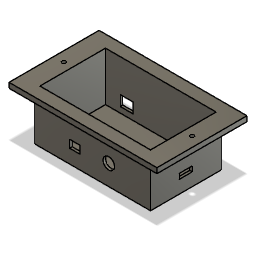
Casing light game v8 (Autodesk Fusion 360 design; units mm, degrees)
Autodesk Fusion 360 part; units mm, degrees
sketch "Sketch1" plane through (0, 0, 0) normal (0, 1, 0) x (1, 0, 0)
  line L0 (57.15, -34.925) -> (-57.15, -34.925)
  line L1 (-57.15, -34.925) -> (-57.15, 34.925)
  line L2 (-57.15, 34.925) -> (57.15, 34.925)
  line L3 (57.15, 34.925) -> (57.15, -34.925)
  line L4 (57.15, -34.925) -> (-57.15, 34.925) construction
  line L5 (-57.15, -34.925) -> (57.15, 34.925) construction
  dimension "d1" = 114.3
  dimension "d2" = 69.85
  constraint horizontal L0
  constraint perpendicular L0 L1
  constraint parallel L0 L2
  constraint parallel L1 L3
  constraint coincident L4 origin
  constraint coincident L5 origin
  measures "d1" distance of L1.end L2.end
  measures "d2" distance of L0.end L1.end
extrude "Extrude1" add sketch "Sketch1" along normal blind 44.45
sketch "Sketch10" plane through (0, 44.45, 0) normal (0, 1, 0) x (-1, 0, 0)
  line L0 (-57.15, -34.925) -> (57.15, -34.925)
  line L1 (57.15, -34.925) -> (57.15, 34.925)
  line L2 (57.15, 34.925) -> (-57.15, 34.925)
  line L3 (-57.15, 34.925) -> (-57.15, -34.925)
  line L4 (-73.025, 44.45) -> (73.025, 44.45)
  line L5 (73.025, 44.45) -> (73.025, -44.45)
  line L6 (73.025, -44.45) -> (-73.025, -44.45)
  line L7 (-73.025, -44.45) -> (-73.025, 44.45)
  line L8 (-73.025, 44.45) -> (73.025, -44.45) construction
  line L9 (73.025, 44.45) -> (-73.025, -44.45) construction
  dimension "d55" = 146.05
  dimension "d56" = 88.9
  constraint horizontal L4
  constraint perpendicular L4 L5
  constraint parallel L4 L6
  constraint parallel L5 L7
  constraint coincident L8 origin
  constraint coincident L9 origin
  measures "d55" distance of L5.end L6.end
  measures "d56" distance of L4.end L5.end
extrude "Extrude14" add sketch "Sketch10" along normal blind 5.08 contours L0 L1 L2 L3 | L4 L5 L6 L7
sketch "Sketch11" plane through (0, 49.53, 0) normal (0, 1, 0) x (-1, 0, 0)
  line L0 (-73.025, -44.45) -> (73.025, -44.45)
  line L1 (73.025, -44.45) -> (73.025, 44.45)
  line L2 (73.025, 44.45) -> (-73.025, 44.45)
  line L3 (-73.025, 44.45) -> (-73.025, -44.45)
  line L4 (57.15, -34.925) -> (-57.15, -34.925)
  line L5 (-57.15, -34.925) -> (-57.15, 34.925)
  line L6 (-57.15, 34.925) -> (57.15, 34.925)
  line L7 (57.15, 34.925) -> (57.15, -34.925)
  line L8 (63.5, -38.1) -> (-63.5, -38.1)
  line L9 (-63.5, -38.1) -> (-63.5, 38.1)
  line L10 (-63.5, 38.1) -> (63.5, 38.1)
  line L11 (63.5, 38.1) -> (63.5, -38.1)
  line L12 (63.5, -38.1) -> (-63.5, 38.1) construction
  line L13 (-63.5, -38.1) -> (63.5, 38.1) construction
  dimension "d61" = 127
  dimension "d62" = 76.2
  constraint horizontal L8
  constraint perpendicular L8 L9
  constraint parallel L8 L10
  constraint parallel L9 L11
  constraint coincident L12 origin
  constraint coincident L13 origin
  measures "d61" distance of L8.start L8.end
  measures "d62" distance of L8.start L10.end
sketch "Sketch27" plane through (0, 49.53, 0) normal (0, 1, 0) x (-1, 0, 0)
  line L0 (-73.025, -44.45) -> (73.025, -44.45)
  line L1 (73.025, -44.45) -> (73.025, 44.45)
  line L2 (73.025, 44.45) -> (-73.025, 44.45)
  line L3 (-73.025, 44.45) -> (-73.025, -44.45)
  line L4 (57.15, -34.925) -> (-57.15, -34.925)
  line L5 (-57.15, -34.925) -> (-57.15, 34.925)
  line L6 (-57.15, 34.925) -> (57.15, 34.925)
  line L7 (57.15, 34.925) -> (57.15, -34.925)
  line L8 (-54.61, 32.385) -> (54.61, 32.385)
  line L9 (54.61, 32.385) -> (54.61, -32.385)
  line L10 (54.61, -32.385) -> (-54.61, -32.385)
  line L11 (-54.61, -32.385) -> (-54.61, 32.385)
  dimension "d89" = 2.54
extrude "Extrude22" cut sketch "Sketch27" against normal blind 48.26 contours L8 L9 L10 L11
sketch "Sketch28" plane through (0, 49.53, 0) normal (0, 1, 0) x (-1, 0, 0)
  line L0 (54.61, 32.385) -> (54.61, -32.385)
  line L1 (54.61, -32.385) -> (-54.61, -32.385)
  line L2 (-54.61, -32.385) -> (-54.61, 32.385)
  line L3 (-54.61, 32.385) -> (54.61, 32.385)
  line L4 (-73.025, -44.45) -> (73.025, -44.45)
  line L5 (73.025, -44.45) -> (73.025, 44.45)
  line L6 (73.025, 44.45) -> (-73.025, 44.45)
  line L7 (-73.025, 44.45) -> (-73.025, -44.45)
  circle A0 centre (63.373, 0) radius 1.905
  line L8 (0, 0) -> (0, 7.62)
  circle A1 centre (-63.373, 0) radius 1.905
  dimension "d92" = 3.81
  dimension "d93" = 9.652
  constraint coincident L8.start origin
  constraint perpendicular L1 L8
  constraint symmetric A0 L8 A1
  measures "d92" diameter of A0
  measures "d93" distance of L5 A0.centre
extrude "Extrude23" cut sketch "Sketch28" against normal blind 38.1 contours A0 | A1
sketch "Sketch29" plane through (0, 0, 34.925) normal (0, 0, 1) x (1, 0, 0)
  line L0 (-57.15, 0) -> (57.15, 0)
  line L1 (57.15, 0) -> (57.15, 44.45)
  line L2 (57.15, 44.45) -> (-57.15, 44.45)
  line L3 (-57.15, 44.45) -> (-57.15, 0)
  line L4 (-22.698, 21.1911) -> (-12.538, 21.1911)
  line L5 (-12.538, 21.1911) -> (-12.538, 13.5711)
  line L6 (-12.538, 13.5711) -> (-22.698, 13.5711)
  line L7 (-22.698, 13.5711) -> (-22.698, 21.1911)
  circle A0 centre (15.9589, 19.9606) radius 5.715
  dimension "d96" = 10.16
  dimension "d97" = 7.62
  dimension "d98" = 11.43
  constraint horizontal L4
  constraint vertical L5
  constraint horizontal L6
  constraint vertical L7
  measures "d96" distance of L4.start L4.end
  measures "d97" distance of L4.start L6.end
  measures "d98" diameter of A0
sketch "Sketch30" plane through (0, 0, -34.925) normal (0, 0, -1) x (-1, 0, 0)
  line L0 (-57.15, 0) -> (57.15, 0)
  line L1 (57.15, 0) -> (57.15, 44.45)
  line L2 (57.15, 44.45) -> (-57.15, 44.45)
  line L3 (-57.15, 44.45) -> (-57.15, 0)
  line L4 (40.0812, 6.9441) -> (27.3812, 6.9441)
  line L5 (27.3812, 6.9441) -> (27.3812, 17.1041)
  line L6 (27.3812, 17.1041) -> (40.0812, 17.1041)
  line L7 (40.0812, 17.1041) -> (40.0812, 6.9441)
  dimension "d114" = 12.7
  dimension "d115" = 10.16
  constraint horizontal L4
  constraint vertical L5
  constraint horizontal L6
  constraint vertical L7
  measures "d114" distance of L4.start L4.end
  measures "d115" distance of L4.start L6.end
sketch "Sketch31" plane through (57.15, 0, 0) normal (1, 0, 0) x (0, 0, -1)
  line L0 (-34.925, 0) -> (34.925, 0)
  line L1 (34.925, 0) -> (34.925, 44.45)
  line L2 (34.925, 44.45) -> (-34.925, 44.45)
  line L3 (-34.925, 44.45) -> (-34.925, 0)
  line L4 (6.35, 12.7) -> (-6.35, 12.7)
  line L5 (-6.35, 12.7) -> (-6.35, 17.78)
  line L6 (-6.35, 17.78) -> (6.35, 17.78)
  line L7 (6.35, 17.78) -> (6.35, 12.7)
  line L8 (6.35, 12.7) -> (-6.35, 17.78) construction
  line L9 (-6.35, 12.7) -> (6.35, 17.78) construction
  point P0 (0, 15.24)
  dimension "d101" = 12.7
  dimension "d102" = 5.08
  constraint horizontal L4
  constraint perpendicular L4 L5
  constraint parallel L4 L6
  constraint parallel L5 L7
  constraint coincident L8 P0
  constraint coincident L9 P0
  measures "d101" distance of L5.end L6.end
  measures "d102" distance of L4.end L5.end
extrude "Extrude24" cut sketch "Sketch29" against normal blind 40.64 contours L4 L5 L6 L7 | A0
extrude "Extrude25" cut sketch "Sketch30" against normal blind 33.02 contours L4 L5 L6 L7
extrude "Extrude26" cut sketch "Sketch31" against normal blind 33.02 contours L4 L5 L6 L7
sketch "Sketch32" plane through (0, 1.27, 0) normal (0, 1, 0) x (-1, 0, 0)
  line L0 (-54.61, -32.385) -> (54.61, -32.385)
  line L1 (54.61, -32.385) -> (54.61, 32.385)
  line L2 (54.61, 32.385) -> (-54.61, 32.385)
  line L3 (-54.61, 32.385) -> (-54.61, -32.385)
  circle A0 centre (43.18, -5.08) radius 1.1938
  line L4 (43.18, -5.08) -> (-30.0482, -5.08)
  circle A1 centre (-30.0482, -5.08) radius 1.1938
  dimension "d109" = 2.3876
  dimension "d110" = 73.2282
  dimension "d111" = 2.3876
  constraint coincident A0.centre L4.start
  constraint horizontal L4
  constraint coincident L4.end A1.centre
  measures "d109" diameter of A0
  measures "d110" distance of A0.centre L4.end
  measures "d111" diameter of A1
extrude "Extrude27" cut sketch "Sketch32" against normal blind 10.16 contours A0 | A1
